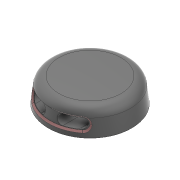
# Autodesk Inventor part: bovenkant rplidar
Saved by Autodesk Inventor 2020.3 (Build 243373000, 373)
## iProperties
Created: 2020-09-30
Part Number: bovenkant rplidar
Material: Acetal Resin, Black
Document SubType Name: Modeling
Designer: Svend
Density: 1.425 g/cm^3
Appearance: Smooth - Black
Author: Svend
Autodesk Inventor part; units mm, degrees
ref_plane "YZ Plane" through (0, 0, 0) normal (1, 0, 0) x (0, 1, 0)
ref_plane "XZ Plane" through (0, 0, 0) normal (0, 1, 0) x (-1, 0, 0)
sketch "Sketch1" plane through (0, 0, 0) normal (0, 0, 1) x (1, 0, 0)
  line L0 (0, 0) -> (36.25, 0)
  line L1 (36.25, 0) -> (34, 21.5)
  line L2 (34, 21.5) -> (0, 21.5)
  line L3 (0, 21.5) -> (0, 0)
  dimension "d0" = 36.25
  dimension "d1" = 34
  dimension "d2" = 21.5
  constraints: 8 end point, 2 horizontal, 1 coincident, 1 perpendicular
  measures "d0" distance of L0.start L0.end
  measures "d1" distance of L1.end L2.end
  measures "d2" distance between parallel lines of L0 L2
revolve "Revolution1" add sketch "Sketch1" angle 360 about axis through (0, 21.5, 0) along (0, -1, 0)
fillet "Fillet1" radius 8 1 edges at (-34, 21.5, 0)
sketch "Sketch2" plane through (0, 0, 0) normal (1, 0, 0) x (0, 1, 0)
  arc A0 (21.5, 26.7935) -> (14.3327, 34.7501) centre (13.5, 26.7935) ccw projected
  line L0 (14.3327, 34.7501) -> (0, 36.25) projected
  arc A1 (20, 26.7935) -> (14.1765, 33.2582) centre (13.5, 26.7935) ccw
  line L1 (14.1765, 33.2582) -> (-0.1561, 34.7581)
  line L2 (5, 34.2186) -> (5, 35.7267)
  line L3 (13.843, 33.2845) -> (14, 34.7849)
  line L4 (0, 36.25) -> (0, -36.25) projected
  line L5 (-4.7929, 0) -> (27.6644, 0) projected
  point P0 (0, 0)
  point P1 (0, 34.7418)
  point P2 (13.8439, 33.293)
  dimension "d5" = 1.5
  dimension "d6" = 1.5
  dimension "d9" = 5
  dimension "d25" = 9
  constraints: 6 end point, 3 point on circle, 3 point on line, 2 parallel, 1 centre point, 1 perpendicular
  measures "d5" radial gap between concentric circles of A0 A1
  measures "d6" distance between parallel lines of L0 L1
  measures "d9" distance from line of L4 L2.end
  measures "d25" distance from line of L2 L3.end
revolve "Revolution2" cut sketch "Sketch2" angle 90 mid plane about axis through (0, -10, 0) along (0, 1, 0) contours L3 L1 L2 L0
fillet "Fillet2" radius 4.6 4 edges at (24.0692, 13.9219, 24.0692) (24.7294, 5, 24.7294) (-24.7294, 5, 24.7294) (-24.0692, 13.9219, 24.0692)
chamfer "Chamfer1" distance 1.3 angle 45 5 edges at (23.9134, 12.4369, 25.4862) (24.3411, 6.5929, 25.9235) (0, 5, 35.7267) (-24.3411, 6.5929, 25.9235) (-23.9134, 12.4369, 25.4862)
ref_plane "Work Plane1" through (0, 0, 11) normal (0, 0, 1) x (1, 0, 0)
sketch "Sketch3" plane through (0, 0, 11) normal (0, 0, 1) x (1, 0, 0)
  line L0 (-20.8724, 5) -> (20.8784, 5) projected
  circle A0 centre (-18.8558, 9.4323) radius 4.25
  circle A1 centre (-9.3558, 9.4323) radius 4.25
  line L1 (-18.8558, 13.6823) -> (-9.3558, 13.6823)
  line L2 (-9.3558, 5.1823) -> (-18.8558, 5.1823)
  line L3 (-14.1058, 5.1823) -> (-14.1058, 5) construction
  line L4 (0, 16.3647) -> (0.003, 5) construction
  circle A2 centre (18.8594, 9.4422) radius 4.25
  circle A3 centre (9.3594, 9.4372) radius 4.25
  line L5 (18.8572, 13.6922) -> (9.3572, 13.6872)
  line L6 (9.3616, 5.1872) -> (18.8616, 5.1922)
  line L7 (-20.2657, 13.8647) -> (20.2574, 13.8647) projected
  line L8 (-14.1058, 13.6823) -> (-14.1058, 13.8647) construction
  point P0 (0, 0)
  point P1 (-23.1058, 9.4323)
  point P2 (-5.1058, 9.4323)
  point P3 (18.8572, 13.6922)
  point P4 (9.3572, 13.6872)
  point P5 (14.1116, 5.1897)
  point P6 (12.3577, 12.6513)
  point P7 (23.1094, 9.4444)
  point P8 (5.1094, 9.435)
  point P9 (-19.8269, 5)
  point P10 (-24.5662, 0)
  point P11 (24.5662, 0)
  point P12 (19.8269, 5)
  dimension "d17" = 8.5
  dimension "d20" = 5
  dimension "d21" = 18
  constraints: 12 end point, 12 point on circle, 9 symmetric about line, 4 centre point, 4 tangent, 3 horizontal alignment, 3 midpoint, 2 point on line, 1 collinear, 1 equal radius, 1 perpendicular, 1 vertical, 9 other
  measures "d17" diameter of A0
  measures "d20" horizontal distance of point (-23.856, 9.6) A0.centre
  measures "d21" distance of point (-5.106, 9.432) point (-23.106, 9.432)
extrude "Extrusion2" cut sketch "Sketch3" along normal through all
fillet "Fillet3" radius 0.2 8 edges at (-14.2849, 13.6823, 30.0914) (-5.1061, 9.4848, 33.3607) (-14.2735, 5.1823, 31.0785) (-23.1014, 9.2392, 24.6388) (14.2863, 13.6898, 30.0899) (23.1051, 9.2511, 24.6336) (14.2795, 5.1898, 31.0749) (5.1097, 9.488, 33.3598)
sketch "Sketch4" plane through (0, 0, 0) normal (0, -1, 0) x (1, 0, 0)
  circle A0 centre (0, 0) radius 5
  dimension "d29" = 10
  constraints: 1 centre point, 1 coincident
  measures "d29" diameter of A0
extrude "Extrusion3" cut sketch "Sketch4" against normal blind 5
chamfer "Chamfer2" distance 0.5 angle 45 1 edges at (-36.25, 0, 0)
body "Solid1"
